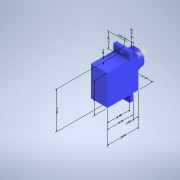
# Autodesk Inventor part: servo_motor
Saved by Autodesk Inventor 2022.1 (Build 261234000, 234)
## iProperties
Created: 2021-08-02
Part Number: servo_motor
Material: Nylon 6/6
Document SubType Name: Modeling
Designer: nakai
Density: 1.13 g/cm^3
Appearance: Nylon 6
Author: nakai
Autodesk Inventor part; units mm, degrees
ref_plane "YZ Plane" through (0, 0, 0) normal (1, 0, 0) x (0, 1, 0)
ref_plane "XZ Plane" through (0, 0, 0) normal (0, 1, 0) x (-1, 0, 0)
ref_plane "XY Plane" through (0, 0, 0) normal (0, 0, 1) x (1, 0, 0)
sketch "Sketch3" plane through (0, 0, 0) normal (0, 0, 1) x (1, 0, 0)
  line L0 (0, 0) -> (12.2, 0)
  line L1 (12.2, 0) -> (12.2, -32.5)
  line L2 (12.2, -32.5) -> (0, -32.5)
  line L3 (0, -32.5) -> (0, 0)
  dimension "d11" = 12.2
  dimension "d12" = 32.5
  constraints: 8 end point, 2 parallel, 1 horizontal, 1 perpendicular
  measures "d11" distance of L1.end L2.end
  measures "d12" distance of L0.end L1.end
extrude "Extrusion3" add sketch "Sketch3" along normal blind 2.5
sketch "Sketch4" plane through (0, 0, 2.5) normal (0, 0, 1) x (1, 0, 0)
  line L0 (0, 0) -> (0, -32.5) projected
  line L1 (12.2, -32.5) -> (12.2, 0) projected
  line L2 (0, -5) -> (12.2, -5)
  line L3 (12.2, -5) -> (12.2, -27.5)
  line L4 (12.2, -27.5) -> (0, -27.5)
  line L5 (0, -27.5) -> (0, -5)
  line L6 (12.2, 0) -> (0, 0) projected
  dimension "d15" = 22.5
  dimension "d16" = 5
  constraints: 8 end point, 2 parallel, 2 point on line, 1 horizontal, 1 perpendicular
  measures "d15" distance of L2.end L3.end
  measures "d16" distance between parallel lines of L6 L2
extrude "Extrusion4" add sketch "Sketch4" along normal blind 16.5 contours L2 L1 L4 L0
sketch "Sketch5" plane through (0, 0, 0) normal (0, 0, -1) x (-1, 0, 0)
  line L0 (0, -5) -> (-12.2, -5) projected
  line L1 (-12.2, -27.5) -> (0, -27.5) projected
  line L2 (-12.2, -5) -> (0, -5)
  line L3 (0, -5) -> (0, -27.5)
  line L4 (0, -27.5) -> (-12.2, -27.5)
  line L5 (-12.2, -27.5) -> (-12.2, -5)
  point P0 (0, 0)
  constraints: 8 end point, 2 parallel, 1 horizontal, 1 perpendicular
extrude "Extrusion5" add sketch "Sketch5" along normal blind 4
sketch "Sketch6" plane through (0, 0, 0) normal (0, 0, -1) x (-1, 0, 0)
  circle A0 centre (-6.1, -2.5) radius 1.25
  circle A1 centre (-6.1, -30) radius 1.25
  line L0 (-12.2, -27.5) -> (0, -27.5) projected
  line L1 (-12.2, 0) -> (0, 0) projected
  line L2 (-12.2, -5) -> (-12.2, 0) projected
  line L3 (-12.2, -32.5) -> (-12.2, -27.5) projected
  dimension "d21" = 2.5
  dimension "d22" = 2.5
  dimension "d23" = 2.5
  dimension "d24" = 2.5
  dimension "d25" = 6.1
  dimension "d26" = 6.1
  constraints: 2 centre point
  measures "d21" diameter of A0
  measures "d22" diameter of A1
  measures "d23" distance from line of L0 A1.centre
  measures "d24" distance from line of L1 A0.centre
  measures "d25" distance from line of L2 A0.centre
  measures "d26" distance from line of L3 A1.centre
extrude "Extrusion6" cut sketch "Sketch6" against normal up to surface (2.5 mm away)
sketch "Sketch7" plane through (0, 0, -4) normal (0, 0, -1) x (-1, 0, 0)
  circle A0 centre (-6.1, -11.1) radius 6.1
  line L0 (0, -5) -> (0, -27.5) projected
  line L1 (0, -5) -> (-12.2, -5) projected
  circle A1 centre (-6.1, -16.5) radius 2.8
  line L2 (-12.2, -27.5) -> (0, -27.5) projected
  point P0 (0, 0)
  point P1 (-3.3001, -16.5194)
  point P2 (-8.8999, -16.5194)
  point P3 (-6.1, -5)
  point P4 (0, -11.1)
  dimension "d29" = 6.1
  dimension "d30" = 12.2
  dimension "d33" = 5.6
  dimension "d34" = 11
  constraints: 2 centre point, 1 tangent
  measures "d29" distance from line of L1 A0.centre
  measures "d30" diameter of A0
  measures "d33" diameter of A1
  measures "d34" distance from line of A1.centre L2
extrude "Extrusion7" add sketch "Sketch7" along normal blind 4.5 contours A0 A1 | A1 A0 | A0 A1
sketch "Sketch8" plane through (0, 0, -8.5) normal (0, 0, -1) x (-1, 0, 0)
  arc A0 (-6.1, -5) -> (-12.2, -11.1) centre (-6.1, -11.1) ccw projected
  circle A1 centre (-6.1, -11.1) radius 2.5
  point P0 (0, 0)
  dimension "d35" = 5
  constraints: 1 centre point, 1 coincident
  measures "d35" diameter of A1
extrude "Extrusion8" add sketch "Sketch8" along normal blind 5
body "Solid2"
